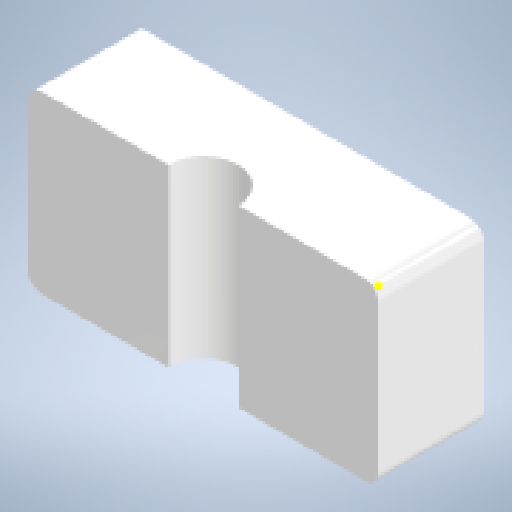
# Autodesk Inventor part: TrittUT
Saved by Autodesk Inventor 2024.4 (Build 284460000, 460)
## iProperties
Created: 2026-01-10
Part Number: TrittUT
Material: PVC, hart
Description: TrittUT
Document SubType Name: Modeling
Designer: Philf
Mass: 180.759 g
Surface Area: 204.743 cm^2
Volume: 140.123 cm^3
Density: 1.29 g/cm^3
Appearance: Glatt - Weiß
Masse[kg]: 0,150 kg
breite: 50,000 mm
länge: 100,000 mm
radius: 4,000 mm
Author: Philf
Autodesk Inventor part; units mm, degrees
ref_plane "YZ Plane" through (0, 0, 0) normal (1, 0, 0) x (0, 1, 0)
ref_plane "XZ Plane" through (0, 0, 0) normal (0, 1, 0) x (-1, 0, 0)
ref_plane "XY Plane" through (0, 0, 0) normal (0, 0, 1) x (1, 0, 0)
sketch "Skizze2" plane through (0, 0, 0) normal (0, 1, 0) x (-1, 0, 0)
  line L0 (0, -4) -> (0, -46)
  line L1 (4, -50) -> (96, -50)
  line L2 (100, -46) -> (100, -4)
  line L3 (96, 0) -> (4, 0)
  arc A0 (100, -4) -> (96, 0) centre (96, -4) ccw
  arc A1 (96, -50) -> (100, -46) centre (96, -46) ccw
  arc A2 (0, -46) -> (4, -50) centre (4, -46) ccw
  arc A3 (4, 0) -> (0, -4) centre (4, -4) ccw
  point P0 (0, 0)
  point P1 (0, -50)
  point P2 (100, -50)
  point P3 (100, 0)
  dimension "breite" = 50
  dimension "länge" = 100
  dimension "d11" = 50
  dimension "radius" = 4
  constraints: 8 end point, 8 point on circle, 8 point on line, 8 tangent, 4 centre point, 3 equal radius, 2 perpendicular, 1 vertical
  measures "breite" distance of point (0, 0) point (0, -50)
  measures "länge" distance of point (0, -50) point (100, -50)
  measures "d11" distance of point (100, -50) point (100, 0)
  measures "radius" radius of A0
extrude "Extrusion2" add sketch "Skizze2" along normal blind 30
sketch "Skizze4" plane through (-96, 0, 0) normal (0, 0, 1) x (1, 0, 0)
  point P0 (96, 0)
sketch "Skizze5" plane through (-96, 0, 0) normal (0, 0, 1) x (1, 0, 0)
  line L0 (0, 0) -> (0, 30) projected
  line L1 (0, 0) -> (46, 0)
  line L2 (92, 0) -> (0, 0) projected
  circle A0 centre (46, 0) radius 10
  point P0 (96, 0)
  dimension "d15" = 20
  constraints: 2 end point, 1 centre point, 1 coincident, 1 midpoint
  measures "d15" diameter of A0
extrude "Extrusion3" cut sketch "Skizze5" against normal through all
sketch "Skizze6" plane through (0, 0, 0) normal (0, -1, 0) x (1, 0, 0)
  line L0 (0, 0) -> (0, -10)
  line L1 (0, -4) -> (0, -46) projected
  line L2 (0, -10) -> (-15, -10)
  line L3 (-15, -10) -> (-85, -10)
  line L4 (-85, -10) -> (-85, -40)
  line L5 (-85, -40) -> (-15, -40)
  dimension "d18" = 10
  dimension "d19" = 15
  dimension "d20" = 70
  dimension "d21" = 30
  dimension "d22" = 70
  constraints: 10 end point, 3 perpendicular, 2 point on line
  measures "d18" distance of L0.start L0.end
  measures "d19" distance of L0.end L2.end
  measures "d20" distance of L2.end L3.end
  measures "d21" distance of L3.end L4.end
  measures "d22" distance of L4.end L5.end
hole "Bohrung1" at (-15, 0, -40) at (-15, 0, -10) at (-85, 0, -40) at (-85, 0, -10) direction (0, 1, 0) diameter 4.134 end through all thread size "M5x0.8" class "6H" standard "ISO Metric profile"
equation "\"d11\" = breite"
equation "\"d15\" = durchmesser"
equation "\"durchmesser\" = 20"
